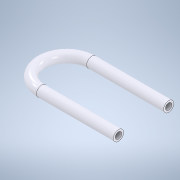
# Autodesk Inventor part: Manguera
Saved by Autodesk Inventor 2020.2 (Build 242310000, 310)
## iProperties
Created: 2021-03-10
Part Number: Manguera
Material: Generic
Document SubType Name: Modeling
Designer: JK
Density: 1 g/cm^3
Appearance: Default
Author: JK
Autodesk Inventor part; units mm, degrees
ref_plane "XZ Plane" through (0, 0, 0) normal (0, 1, 0) x (-1, 0, 0)
ref_plane "XY Plane" through (0, 0, 0) normal (0, 0, 1) x (1, 0, 0)
sketch "Sketch1" plane through (0, 0, 0) normal (0, 1, 0) x (-1, 0, 0)
  arc A0 (0, -19.575) -> (0, 19.575) centre (0, 0) ccw
  line L0 (0, 19.575) -> (-60, 19.575)
  line L1 (0, -19.575) -> (-60, -19.575)
  dimension "d0" = 39.15
  dimension "d1" = 60
  constraints: 4 end point, 2 coincident, 2 horizontal, 2 point on circle, 1 centre point, 1 parallel, 1 tangent, 1 vertical alignment
  measures "d0" diameter of A0
  measures "d1" distance of L0.start L0.end
ref_plane "Work Plane1" through (60, 0, 19.575) normal (1, 0, 0) x (0, 1, 0)
sketch "Sketch2" plane through (60, 0, 19.575) normal (1, 0, 0) x (0, 1, 0)
  circle A0 centre (0, 0) radius 4
  circle A1 centre (0, 0) radius 2.5
  point P0 (0, -19.575)
  dimension "d2" = 8
  dimension "d3" = 5
  constraints: 2 centre point, 1 coincident
  measures "d2" diameter of A0
  measures "d3" diameter of A1
sweep "Sweep1" add profiles "Sketch2" path "Sketch1" path curves L0 A0 L1
body "Solid1"
